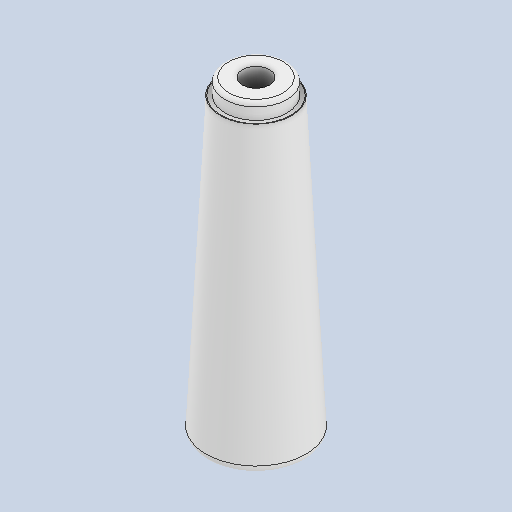
# Autodesk Inventor part: B3OFT4_HF2_kezifuro_HajtokarFogo
Saved by Autodesk Inventor 2023.3 (Build 273359000, 359)
## iProperties
Created: 2023-12-03
Part Number: B3OFT4_HF2_kezifuro_HajtokarFogo
Material: PVC-Piping
Document SubType Name: Modeling
Designer: Csábi-Kis Henrik
Density: 1.4 g/cm^3
Appearance: Smooth - White
Mass: 31.114 g
Surface Area: 88.1696 cm^2
Volume: 22.2243 cm^3
Author: Csábi-Kis Henrik
Autodesk Inventor part; units mm, degrees
ref_plane "YZ Plane" through (0, 0, 0) normal (1, 0, 0) x (0, 1, 0)
ref_plane "XZ Plane" through (0, 0, 0) normal (0, 1, 0) x (-1, 0, 0)
ref_plane "XY Plane" through (0, 0, 0) normal (0, 0, 1) x (1, 0, 0)
derived "B3OFT4_HF2_kezifuro_skeleton.ipt"
sketch "Sketch1" plane through (0, 0, 0) normal (0, 0, 1) x (1, 0, 0)
  line L0 (-14, 0) -> (14, 0) construction
  line L1 (0, 14) -> (0, -14) construction
  line L2 (-43.5, -15) -> (43.5, -15)
  line L3 (43.5, -15) -> (43.5, 15)
  line L4 (43.5, 15) -> (-43.5, 15)
  line L5 (-43.5, 15) -> (-43.5, -15)
  line L6 (-43.5, -15) -> (43.5, 15) construction
  line L7 (43.5, -15) -> (-43.5, 15) construction
  line L8 (-49.5, 21) -> (49.5, 21)
  line L9 (49.5, 21) -> (49.5, -21)
  line L10 (49.5, -21) -> (-49.5, -21)
  line L11 (-49.5, -21) -> (-49.5, 21)
  point P0 (0, 0)
sketch "Sketch2" plane through (0, 0, 0) normal (0, 1, 0) x (-1, 0, 0)
  line L0 (0, -75.2785) -> (0, 75.2785) construction
  line L1 (-69.3, 0) -> (69.3, 0) construction
  line L2 (43.5, -11) -> (-43.5, -11)
  line L3 (-43.5, -11) -> (-43.5, 11)
  line L4 (-43.5, 11) -> (43.5, 11)
  line L5 (43.5, 11) -> (43.5, -11)
  line L6 (43.5, -11) -> (-43.5, 11) construction
  line L7 (-43.5, -11) -> (43.5, 11) construction
  line L8 (22.5, 30.8) -> (-22.5, 30.8)
  line L9 (-43.5, 11) -> (-49.5, 11)
  line L10 (-49.5, 11) -> (-49.5, 0) construction
  arc A0 (-22.5, 30.8) -> (-49.5, 11) centre (-22.5, 2.4909) ccw
  line L11 (43.5, 11) -> (49.5, 11)
  arc A1 (49.5, 11) -> (22.5, 30.8) centre (22.5, 2.4909) ccw
  point P0 (43.5, 0)
  point P1 (43.5, 0)
  point P2 (43.5, 0)
  point P3 (-43.5, 0)
  point P4 (-43.5, 0)
  point P5 (-43.5, 0)
  point P6 (0, 0)
  point P7 (-49.5, 0)
  point P8 (49.5, 0)
  point P9 (49.5, 0)
  point P10 (49.5, 0)
sketch "Sketch3" plane through (0, 13, 0) normal (0, 1, 0) x (-1, 0, 0)
  line L0 (-69.3, 0) -> (69.3, 0) construction
  circle A0 centre (16.7, 0) radius 5
  circle A1 centre (-14.1, 0) radius 5
  circle A2 centre (-14.1, 0) radius 6.5
  point P0 (43.5, 0)
  point P1 (43.5, 0)
  point P2 (43.5, 0)
  point P3 (-43.5, 0)
  point P4 (-43.5, 0)
  point P5 (-43.5, 0)
sketch "Sketch4" plane through (0, 23, 0) normal (0, 1, 0) x (-1, 0, 0)
  circle A0 centre (16.7, 0) radius 5
  circle A1 centre (-14.1, 0) radius 5
sketch "Sketch5" plane through (0, -14.5, 0) normal (0, 1, 0) x (-1, 0, 0)
  circle A0 centre (16.7, 0) radius 5
  circle A1 centre (-14.1, 0) radius 5
sketch "Sketch6" plane through (0, -25, 0) normal (0, 1, 0) x (-1, 0, 0)
  circle A0 centre (16.7, 0) radius 5
  circle A1 centre (-14.1, 0) radius 5
sketch "Sketch7" plane through (0, -43, 0) normal (0, 1, 0) x (-1, 0, 0)
  line L0 (13.5246, -5.5) -> (10.3491, 0)
  line L1 (10.3491, 0) -> (13.5246, 5.5)
  line L2 (13.5246, 5.5) -> (19.8754, 5.5)
  line L3 (19.8754, 5.5) -> (23.0509, 0)
  line L4 (23.0509, 0) -> (19.8754, -5.5)
  line L5 (19.8754, -5.5) -> (13.5246, -5.5)
  point P0 (16.7, 0)
  point P1 (16.7, 0)
sketch "Sketch8" plane through (-66.5, 0, 0) normal (1, 0, 0) x (0, 1, 0)
  circle A0 centre (0, 0) radius 5
sketch "Sketch9" plane through (43.5, 0, 11) normal (0, 0, 1) x (-1, 0, 0)
  line L0 (264.4, 0) -> (-116.4, 0) construction
  line L1 (43.5, -42) -> (43.5, 91) construction
  circle A0 centre (97.5, 0) radius 2.5
  circle A1 centre (-10.5, 0) radius 2.5
  point P0 (43.5, 0)
sketch "Sketch10" plane through (42.5, 0, 0) normal (1, 0, 0) x (0, 1, 0)
  circle A0 centre (0, 0) radius 5
sketch "Sketch11" plane through (105.5, 0, 0) normal (1, 0, 0) x (0, 1, 0)
  circle A0 centre (0, 0) radius 12
  circle A1 centre (0, 0) radius 7
sketch "Sketch12" plane through (99.5, 0, 0) normal (1, 0, 0) x (0, 1, 0)
  circle A0 centre (0, 0) radius 12
  circle A1 centre (0, 0) radius 5
sketch "Sketch13" plane through (0, 0, 0) normal (0, 0, 1) x (1, 0, 0)
  line L0 (-16.7, 23) -> (-16.7, -43)
  line L1 (14.1, 23) -> (14.1, -25)
  circle A0 centre (-16.7, 2.5) radius 1.5
  circle A1 centre (14.1, 3.5) radius 1.5
  line L2 (105.5, 0) -> (30, 0)
  circle A2 centre (39, 0) radius 1.5
  line L3 (75.5, 0) -> (75.5, 15)
  line L4 (-66.5, 0) -> (-166.5, 0)
  line L5 (-11.7, -25) -> (-21.7, -25)
  line L6 (-16.7, -36) -> (-3.8491, -36)
  point P0 (42.5, 0)
  point P1 (-16.7, -27)
  point P2 (-16.7, -25)
  point P3 (-10.3491, -43)
sketch "Sketch14" plane through (30, 0, 0) normal (1, 0, 0) x (0, 1, 0)
  circle A0 centre (0, 0) radius 5
sketch "Sketch15" plane through (75.5, 15, 0) normal (0, 1, 0) x (-1, 0, 0)
  circle A0 centre (0, 0) radius 4
sketch "Sketch17" plane through (-16.7, -27, 0) normal (0, 1, 0) x (-1, 0, 0)
  circle A0 centre (0, 0) radius 11.5
  line L0 (0, 0) -> (100, 0)
  circle A1 centre (100, 0) radius 8.5
  circle A2 centre (100, 0) radius 3.5
sketch "Sketch18" plane through (0, 0, 0) normal (0, 0, 1) x (1, 0, 0)
  line L0 (-116.7, -27) -> (-116.7, -36)
  circle A0 centre (-116.7, -31.5) radius 1.5
  line L1 (-116.7, -36) -> (-116.7, -72)
sketch "Sketch19" plane through (-116.7, -72, 0) normal (0, 1, 0) x (-1, 0, 0)
  circle A0 centre (0, 0) radius 3.5
  circle A1 centre (0, 0) radius 7
sketch "Sketch20" plane through (-3.8491, -36, 0) normal (1, 0, 0) x (0, 1, 0)
  circle A0 centre (0, 0) radius 3
sketch "Sketch21" plane through (-16.7, -36, 0) normal (0, 1, 0) x (-1, 0, 0)
  circle A0 centre (0, 0) radius 5
sketch "Sketch22" plane through (-166.5, 0, 0) normal (1, 0, 0) x (0, 1, 0)
  circle A0 centre (0, 0) radius 9
  point P0 (0, 0)
ref_plane "Work Plane1" through (0, 13, 0) normal (0, 1, 0) x (-1, 0, 0)
ref_plane "Work Plane2" through (0, 23, 0) normal (0, 1, 0) x (-1, 0, 0)
ref_plane "Work Plane3" through (0, -14.5, 0) normal (0, 1, 0) x (-1, 0, 0)
ref_plane "Work Plane4" through (0, -25, 0) normal (0, 1, 0) x (-1, 0, 0)
ref_plane "Work Plane5" through (0, -43, 0) normal (0, 1, 0) x (-1, 0, 0)
ref_plane "Work Plane6" through (-66.5, 0, 0) normal (1, 0, 0) x (0, 1, 0)
ref_plane "Work Plane7" through (43.5, 0, 11) normal (0, 0, 1) x (-1, 0, 0)
ref_plane "Work Plane8" through (42.5, 0, 0) normal (1, 0, 0) x (0, 1, 0)
ref_plane "Work Plane9" through (105.5, 0, 0) normal (1, 0, 0) x (0, 1, 0)
ref_plane "Work Plane10" through (99.5, 0, 0) normal (1, 0, 0) x (0, 1, 0)
ref_plane "Work Plane11" through (30, 0, 0) normal (1, 0, 0) x (0, 1, 0)
ref_plane "Work Plane12" through (75.5, 15, 0) normal (0, 1, 0) x (-1, 0, 0)
ref_plane "Work Plane15" through (-116.7, -72, 0) normal (0, 1, 0) x (-1, 0, 0)
ref_plane "Work Plane16" through (-3.8491, -36, 0) normal (1, 0, 0) x (0, 1, 0)
ref_plane "Work Plane17" through (-16.7, -36, 0) normal (0, 1, 0) x (-1, 0, 0)
ref_plane "Work Plane20" through (0, -13.5, 0) normal (0, 1, 0) x (-1, 0, 0)
ref_plane "Work Plane21" through (0, -1.5, 0) normal (0, 1, 0) x (-1, 0, 0)
ref_plane "Work Plane22" through (37, 0, 0) normal (1, 0, 0) x (0, 1, 0)
sketch "Sketch23" plane through (0, 0, 0) normal (0, 0, 1) x (1, 0, 0)
  line L0 (-116.7, -36) -> (-116.7, -72) construction
  line L1 (-125.7, -36) -> (-107.7, -36)
  line L2 (-107.7, -36) -> (-103.7, -116)
  line L3 (-103.7, -116) -> (-129.7, -116)
  line L4 (-129.7, -116) -> (-125.7, -36)
  line L5 (-116.7, -36) -> (-116.7, -116)
  line L6 (-107.7, -36) -> (-108.7, -36)
  line L7 (-108.7, -36) -> (-108.7, -40)
  line L8 (-108.7, -40) -> (-107.7, -40)
  line L9 (-107.7, -40) -> (-107.7, -36)
  line L10 (-107.7, -40) -> (-107.5005, -39.99)
  dimension "d1" = 26
  dimension "d2" = 18
  dimension "d3" = 80
  dimension "d4" = 1
  dimension "d7" = 4
  constraints: 20 end point, 3 parallel, 2 horizontal, 2 midpoint, 2 perpendicular, 1 point on line, 1 other
  measures "d1" distance of L2.end L3.end
  measures "d2" distance of L1.start L1.end
  measures "d3" distance between parallel lines of L1 L3
  measures "d4" distance of L7.end L8.end
  measures "d7" distance of L6.end L7.end
revolve "Revolution1" add sketch "Sketch23" angle 360 about axis through (-116.7, -36, 0) along (0, -1, 0) contours L1 L7 L8 L10 L2 L3 L5
sketch "Sketch24" plane through (0, 0, 0) normal (0, 0, 1) x (1, 0, 0)
  line L0 (-109.7, -72) -> (-123.7, -72) projected
  line L1 (-129.7, -116) -> (-103.7, -116) projected
  line L2 (-123.7, -72) -> (-116.7, -72)
  line L3 (-116.7, -72) -> (-116.7, -116)
  line L4 (-116.7, -116) -> (-123.7, -116)
  line L5 (-123.7, -116) -> (-123.7, -72)
  constraints: 8 end point, 2 midpoint, 2 parallel, 1 horizontal, 1 perpendicular
revolve "Revolution2" cut sketch "Sketch24" angle 360 about axis through (-116.7, -36, 0) along (0, -1, 0)
extrude "Extrusion1" cut sketch "Sketch17" against normal through all contours A2
fillet "Fillet1" radius 1 1 edges at (-124.7, -36, 0)
fillet "Fillet2" radius 2 2 edges at (-129.7, -116, 0) (-109.7, -116, 0)
ref_plane "Work Plane14" through (-16.7, -27, 0) normal (0, 1, 0) x (-1, 0, 0)
ref_plane "Work Plane19" through (-166.5, 0, 0) normal (1, 0, 0) x (0, 1, 0)
body "Solid1"
